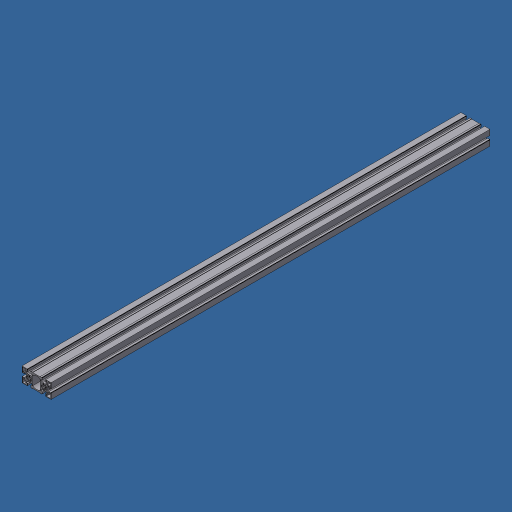
# Autodesk Inventor part: BAR, EXTRUDED ALUM, 45MMX90MM, BOSCH
Saved by Autodesk Inventor 2024.3 (Build 283343000, 343)
## iProperties
Manager: _
Category: _
Control State: 0
Master: False
Checked Out: False
Created: 2019-07-31
Checked By: 00
User Status: Work In Process
Material: Aluminum, 6061-T6
Description: BAR, EXTRUDED ALUM, 45MMX90MM, BOSCH
Document SubType Name: Modeling
Designer: -
Engr Approved By: R
Density: 2.71 g/cm^3
Mass: 5427.32 g
Surface Area: 13744.3 cm^2
Volume: 2002.7 cm^3
Mfg Approved By: -
Part Number: BAR, EXTRUDED ALUM, 45MMX90MM, BOSCH
Appearance: Aluminum (Flat)
Shininess: 64.0
Angle Display Precision: 2
Document Length Units: 11269
Document Angle Units: 11279
Document Time Units: 11290
Document Mass Units: 11283
Document Length Units Precision: 3
Document Angle Units Precision: 2
ILogicPurgeVersion: 2.2.20.20
Density: 0.0
Volumn: 0.0
Area: 0.0
PropertySet Name: Model Information
CN_MASS: 15.74
CN_SERVICEABLE: _
CL_runCount: 0
FIRST_DESCRIPTION: _
SECOND_DESCRIPTION: _
THIRD_DESCRIPTION: _
ModelCat: Uncategorized
Revision Number: A
Subject: _
Author: -
Keywords: -
Autodesk Inventor part; units mm, degrees
ref_plane "YZ Plane" through (0, 0, 0) normal (1, 0, 0) x (0, 1, 0)
ref_plane "XZ Plane" through (0, 0, 0) normal (0, 1, 0) x (-1, 0, 0)
ref_plane "XY Plane" through (0, 0, 0) normal (0, 0, 1) x (1, 0, 0)
sketch "Sketch1" plane through (0, 0, 0) normal (0, 0, 1) x (1, 0, 0)
  line L0 (0.8723, 4.7995) -> (0.562, 7.7834)
  line L1 (-0.9902, 4.2192) -> (-2.4189, 6.8572)
  line L2 (-2.4889, 2.9702) -> (-4.8184, 4.8607)
  line L3 (-3.3956, 1.2428) -> (-6.2711, 2.0979)
  line L4 (-3.5722, -0.7001) -> (-6.5561, -1.0105)
  line L5 (-2.9918, -2.5627) -> (-5.6298, -3.9913)
  line L6 (-1.7429, -4.0614) -> (-3.6333, -6.3908)
  line L7 (-0.0155, -4.9681) -> (-0.8706, -7.8436)
  line L8 (1.9274, -5.1447) -> (2.2378, -8.1286)
  line L9 (3.79, -4.5643) -> (5.2187, -7.2023)
  line L10 (5.2887, -3.3153) -> (7.6181, -5.2058)
  line L11 (6.1954, -1.5879) -> (9.0709, -2.443)
  line L12 (6.372, 0.355) -> (9.3559, 0.6654)
  line L13 (5.7916, 2.2176) -> (8.4296, 3.6462)
  line L14 (4.5427, 3.7163) -> (6.4331, 6.0457)
  line L15 (2.8152, 4.6229) -> (3.6704, 7.4985)
  arc A0 (-2.4889, 2.9702) -> (-3.3956, 1.2428) centre (1.3999, -0.1726) ccw
  arc A1 (-3.5722, -0.7001) -> (-2.9918, -2.5627) centre (1.3999, -0.1726) ccw
  arc A2 (-1.7429, -4.0614) -> (-0.0155, -4.9681) centre (1.3999, -0.1726) ccw
  arc A3 (1.9274, -5.1447) -> (3.79, -4.5643) centre (1.3999, -0.1726) ccw
  arc A4 (5.2887, -3.3153) -> (6.1954, -1.5879) centre (1.3999, -0.1726) ccw
  arc A5 (6.372, 0.355) -> (5.7916, 2.2176) centre (1.3999, -0.1726) ccw
  arc A6 (4.5427, 3.7163) -> (2.8152, 4.6229) centre (1.3999, -0.1726) ccw
  arc A7 (0.8723, 4.7995) -> (-0.9902, 4.2192) centre (1.3999, -0.1726) ccw
  arc A8 (8.4296, 3.6462) -> (6.4331, 6.0457) centre (1.3999, -0.1726) ccw
  arc A9 (9.0709, -2.443) -> (9.3559, 0.6654) centre (1.3999, -0.1726) ccw
  arc A10 (5.2187, -7.2023) -> (7.6181, -5.2058) centre (1.3999, -0.1726) ccw
  arc A11 (-0.8706, -7.8436) -> (2.2378, -8.1286) centre (1.3999, -0.1726) ccw
  arc A12 (-5.6298, -3.9913) -> (-3.6333, -6.3908) centre (1.3999, -0.1726) ccw
  arc A13 (-6.2711, 2.0979) -> (-6.5561, -1.0105) centre (1.3999, -0.1726) ccw
  arc A14 (3.6704, 7.4985) -> (0.562, 7.7834) centre (1.3999, -0.1726) ccw
  arc A15 (-2.4189, 6.8572) -> (-4.8184, 4.8607) centre (1.3999, -0.1726) ccw
  line L16 (-5.4014, 9.3274) -> (-1.7226, 9.3274)
  line L17 (4.5224, 9.3274) -> (8.0715, 9.3274)
  line L18 (8.2012, -9.6726) -> (4.5224, -9.6726)
  line L19 (-1.7226, -9.6726) -> (-5.2717, -9.6726)
  line L20 (-8.1001, -6.9739) -> (-8.1001, -3.2951)
  line L21 (-8.1001, 2.9499) -> (-8.1001, 6.499)
  arc A16 (-8.1001, 2.9499) -> (-8.1001, -3.2951) centre (1.3999, -0.1726) ccw
  arc A17 (4.5224, 9.3274) -> (-1.7226, 9.3274) centre (1.3999, -0.1726) ccw
  arc A18 (-1.7226, -9.6726) -> (4.5224, -9.6726) centre (1.3999, -0.1726) ccw
  line L22 (10.3005, 11.4268) -> (10.3005, 15.3274)
  line L23 (10.3005, 15.3274) -> (6.3999, 15.3274)
  line L24 (6.3999, 15.3274) -> (6.3999, 21.3274)
  line L25 (7.3999, 22.3274) -> (40.3999, 22.3274)
  line L26 (23.8999, 22.3274) -> (23.8999, 5.8274)
  line L27 (22.8999, 4.8274) -> (16.8999, 4.8274)
  line L28 (16.8999, 4.8274) -> (16.8999, 8.7281)
  line L29 (16.8999, 8.7281) -> (12.9992, 8.7281)
  line L30 (10.8999, 6.6287) -> (12.9992, 8.7281)
  line L31 (8.0715, 9.3274) -> (10.3005, 11.4268)
  line L32 (12.5715, 11.3425) -> (18.8822, 11.3425)
  line L33 (18.8822, 11.3425) -> (18.8822, 6.7953)
  line L34 (18.8822, 6.7953) -> (21.9064, 6.7953)
  line L35 (21.9064, 6.7953) -> (21.9064, 20.3274)
  line L36 (21.9064, 20.3274) -> (8.3743, 20.3274)
  line L37 (8.3743, 20.3274) -> (8.3743, 17.3032)
  line L38 (8.3743, 17.3032) -> (12.5715, 17.3032)
  line L39 (12.5715, 17.3032) -> (12.5715, 11.3425)
  line L40 (6.3999, 21.3274) -> (7.3999, 21.3274)
  line L41 (7.3999, 21.3274) -> (7.3999, 22.3274)
  line L42 (22.8999, 4.8274) -> (22.8999, 5.8274)
  line L43 (22.8999, 5.8274) -> (23.8999, 5.8274)
  line L44 (-10.1995, 8.7281) -> (-14.1001, 8.7281)
  line L45 (-14.1001, 8.7281) -> (-14.1001, 4.8274)
  line L46 (-14.1001, 4.8274) -> (-20.1001, 4.8274)
  line L47 (-21.1001, 5.8274) -> (-21.1001, 22.3274)
  line L48 (-21.1001, 22.3274) -> (-4.6001, 22.3274)
  line L49 (-3.6001, 21.3274) -> (-3.6001, 15.3274)
  line L50 (-3.6001, 15.3274) -> (-7.5008, 15.3274)
  line L51 (-7.5008, 15.3274) -> (-7.5008, 11.4268)
  line L52 (-5.4014, 9.3274) -> (-7.5008, 11.4268)
  line L53 (-8.1001, 6.499) -> (-10.1995, 8.7281)
  line L54 (-10.1152, 10.9991) -> (-10.1152, 17.3097)
  line L55 (-10.1152, 17.3097) -> (-5.568, 17.3097)
  line L56 (-5.568, 17.3097) -> (-5.568, 20.334)
  line L57 (-5.568, 20.334) -> (-19.1001, 20.334)
  line L58 (-19.1001, 20.334) -> (-19.1001, 6.8019)
  line L59 (-19.1001, 6.8019) -> (-16.0758, 6.8019)
  line L60 (-16.0758, 6.8019) -> (-16.0758, 10.9991)
  line L61 (-16.0758, 10.9991) -> (-10.1152, 10.9991)
  line L62 (-20.1001, 4.8274) -> (-20.1001, 5.8274)
  line L63 (-20.1001, 5.8274) -> (-21.1001, 5.8274)
  line L64 (-3.6001, 21.3274) -> (-4.6001, 21.3274)
  line L65 (-4.6001, 21.3274) -> (-4.6001, 22.3274)
  line L66 (-7.5008, -11.7719) -> (-7.5008, -15.6726)
  line L67 (-7.5008, -15.6726) -> (-3.6001, -15.6726)
  line L68 (-3.6001, -15.6726) -> (-3.6001, -21.6726)
  line L69 (-4.6001, -22.6726) -> (-21.1001, -22.6726)
  line L70 (-21.1001, -22.6726) -> (-21.1001, -6.1726)
  line L71 (-20.1001, -5.1726) -> (-14.1001, -5.1726)
  line L72 (-14.1001, -5.1726) -> (-14.1001, -9.0732)
  line L73 (-14.1001, -9.0732) -> (-10.1995, -9.0732)
  line L74 (-8.1001, -6.9739) -> (-10.1995, -9.0732)
  line L75 (-5.2717, -9.6726) -> (-7.5008, -11.7719)
  line L76 (-9.7717, -11.6876) -> (-16.0824, -11.6876)
  line L77 (-16.0824, -11.6876) -> (-16.0824, -7.1405)
  line L78 (-16.0824, -7.1405) -> (-19.1067, -7.1405)
  line L79 (-19.1067, -7.1405) -> (-19.1067, -20.6726)
  line L80 (-19.1067, -20.6726) -> (-5.5746, -20.6726)
  line L81 (-5.5746, -20.6726) -> (-5.5746, -17.6483)
  line L82 (-5.5746, -17.6483) -> (-9.7717, -17.6483)
  line L83 (-9.7717, -17.6483) -> (-9.7717, -11.6876)
  line L84 (-3.6001, -21.6726) -> (-4.6001, -21.6726)
  line L85 (-4.6001, -21.6726) -> (-4.6001, -22.6726)
  line L86 (-20.1001, -5.1726) -> (-20.1001, -6.1726)
  line L87 (-20.1001, -6.1726) -> (-21.1001, -6.1726)
  line L88 (12.9992, -9.0732) -> (16.8999, -9.0732)
  line L89 (16.8999, -9.0732) -> (16.8999, -5.1726)
  line L90 (16.8999, -5.1726) -> (22.8999, -5.1726)
  line L91 (23.8999, -6.1726) -> (23.8999, -22.6726)
  line L92 (40.3999, -22.6726) -> (7.3999, -22.6726)
  line L93 (6.3999, -21.6726) -> (6.3999, -15.6726)
  line L94 (6.3999, -15.6726) -> (10.3005, -15.6726)
  line L95 (10.3005, -15.6726) -> (10.3005, -11.7719)
  line L96 (8.2012, -9.6726) -> (10.3005, -11.7719)
  line L97 (10.8999, -6.8441) -> (12.9992, -9.0732)
  line L98 (12.9149, -11.3442) -> (12.9149, -17.6548)
  line L99 (12.9149, -17.6548) -> (8.3678, -17.6548)
  line L100 (8.3678, -17.6548) -> (8.3678, -20.6791)
  line L101 (8.3678, -20.6791) -> (21.8999, -20.6791)
  line L102 (21.8999, -20.6791) -> (21.8999, -7.147)
  line L103 (21.8999, -7.147) -> (18.8756, -7.147)
  line L104 (18.8756, -7.147) -> (18.8756, -11.3442)
  line L105 (18.8756, -11.3442) -> (12.9149, -11.3442)
  line L106 (22.8999, -5.1726) -> (22.8999, -6.1726)
  line L107 (22.8999, -6.1726) -> (23.8999, -6.1726)
  line L108 (6.3999, -21.6726) -> (7.3999, -21.6726)
  line L109 (7.3999, -21.6726) -> (7.3999, -22.6726)
  line L110 (46.9274, 4.7995) -> (47.2378, 7.7834)
  line L111 (48.79, 4.2192) -> (50.2187, 6.8572)
  line L112 (50.2887, 2.9702) -> (52.6181, 4.8607)
  line L113 (51.1954, 1.2428) -> (54.0709, 2.0979)
  line L114 (51.372, -0.7001) -> (54.3559, -1.0105)
  line L115 (50.7916, -2.5627) -> (53.4296, -3.9913)
  line L116 (49.5427, -4.0614) -> (51.4331, -6.3908)
  line L117 (47.8152, -4.9681) -> (48.6704, -7.8436)
  line L118 (45.8723, -5.1447) -> (45.562, -8.1286)
  line L119 (44.0098, -4.5643) -> (42.5811, -7.2023)
  line L120 (42.5111, -3.3153) -> (40.1816, -5.2058)
  line L121 (41.6044, -1.5879) -> (38.7289, -2.443)
  line L122 (41.4278, 0.355) -> (38.4439, 0.6654)
  line L123 (42.0082, 2.2176) -> (39.3702, 3.6462)
  line L124 (43.2571, 3.7163) -> (41.3667, 6.0457)
  line L125 (44.9845, 4.6229) -> (44.1294, 7.4985)
  arc A19 (51.1954, 1.2428) -> (50.2887, 2.9702) centre (46.3999, -0.1726) ccw
  arc A20 (50.7916, -2.5627) -> (51.372, -0.7001) centre (46.3999, -0.1726) ccw
  arc A21 (47.8152, -4.9681) -> (49.5427, -4.0614) centre (46.3999, -0.1726) ccw
  arc A22 (44.0098, -4.5643) -> (45.8723, -5.1447) centre (46.3999, -0.1726) ccw
  arc A23 (41.6044, -1.5879) -> (42.5111, -3.3153) centre (46.3999, -0.1726) ccw
  arc A24 (42.0082, 2.2176) -> (41.4278, 0.355) centre (46.3999, -0.1726) ccw
  arc A25 (44.9845, 4.6229) -> (43.2571, 3.7163) centre (46.3999, -0.1726) ccw
  arc A26 (48.79, 4.2192) -> (46.9274, 4.7995) centre (46.3999, -0.1726) ccw
  arc A27 (41.3667, 6.0457) -> (39.3702, 3.6462) centre (46.3999, -0.1726) ccw
  arc A28 (38.4439, 0.6654) -> (38.7289, -2.443) centre (46.3999, -0.1726) ccw
  arc A29 (40.1816, -5.2058) -> (42.5811, -7.2023) centre (46.3999, -0.1726) ccw
  arc A30 (45.562, -8.1286) -> (48.6704, -7.8436) centre (46.3999, -0.1726) ccw
  arc A31 (51.4331, -6.3908) -> (53.4296, -3.9913) centre (46.3999, -0.1726) ccw
  arc A32 (54.3559, -1.0105) -> (54.0709, 2.0979) centre (46.3999, -0.1726) ccw
  arc A33 (47.2378, 7.7834) -> (44.1294, 7.4985) centre (46.3999, -0.1726) ccw
  arc A34 (52.6181, 4.8607) -> (50.2187, 6.8572) centre (46.3999, -0.1726) ccw
  line L126 (53.2012, 9.3274) -> (49.5224, 9.3274)
  line L127 (49.5224, -9.6726) -> (53.0715, -9.6726)
  line L128 (55.8999, -6.9739) -> (55.8999, -3.2951)
  line L129 (55.8999, 2.9499) -> (55.8999, 6.499)
  arc A35 (55.8999, -3.2951) -> (55.8999, 2.9499) centre (46.3999, -0.1726) ccw
  arc A36 (49.5224, 9.3274) -> (43.2774, 9.3274) centre (46.3999, -0.1726) ccw
  arc A37 (43.2774, -9.6726) -> (49.5224, -9.6726) centre (46.3999, -0.1726) ccw
  line L130 (57.9992, 8.7281) -> (61.8999, 8.7281)
  line L131 (63.8756, 10.9991) -> (57.9149, 10.9991)
  line L132 (57.9149, 10.9991) -> (57.9149, 17.3097)
  line L133 (66.8999, 20.334) -> (66.8999, 6.8019)
  line L134 (68.8999, 5.8274) -> (68.8999, 22.3274)
  line L135 (61.8999, 8.7281) -> (61.8999, 4.8274)
  line L136 (61.8999, 4.8274) -> (67.8999, 4.8274)
  line L137 (63.8756, 6.8019) -> (63.8756, 10.9991)
  line L138 (66.8999, 6.8019) -> (63.8756, 6.8019)
  line L139 (67.8999, 5.8274) -> (68.8999, 5.8274)
  line L140 (67.8999, 4.8274) -> (67.8999, 5.8274)
  line L141 (53.3678, 20.334) -> (66.8999, 20.334)
  line L142 (68.8999, 22.3274) -> (52.3999, 22.3274)
  line L143 (51.3999, 15.3274) -> (55.3005, 15.3274)
  line L144 (51.3999, 21.3274) -> (51.3999, 15.3274)
  line L145 (51.3999, 21.3274) -> (52.3999, 21.3274)
  line L146 (53.3678, 17.3097) -> (53.3678, 20.334)
  line L147 (52.3999, 21.3274) -> (52.3999, 22.3274)
  line L148 (57.9149, 17.3097) -> (53.3678, 17.3097)
  line L149 (53.2012, 9.3274) -> (55.3005, 11.4268)
  line L150 (55.3005, 15.3274) -> (55.3005, 11.4268)
  line L151 (55.8999, 6.499) -> (57.9992, 8.7281)
  line L152 (55.3005, -11.7719) -> (55.3005, -15.6726)
  line L153 (57.5715, -17.6483) -> (57.5715, -11.6876)
  line L154 (57.5715, -11.6876) -> (63.8822, -11.6876)
  line L155 (66.9064, -20.6726) -> (53.3743, -20.6726)
  line L156 (52.3999, -22.6726) -> (68.8999, -22.6726)
  line L157 (55.3005, -15.6726) -> (51.3999, -15.6726)
  line L158 (51.3999, -15.6726) -> (51.3999, -21.6726)
  line L159 (53.3743, -17.6483) -> (57.5715, -17.6483)
  line L160 (53.3743, -20.6726) -> (53.3743, -17.6483)
  line L161 (52.3999, -21.6726) -> (52.3999, -22.6726)
  line L162 (51.3999, -21.6726) -> (52.3999, -21.6726)
  line L163 (66.9064, -7.1405) -> (66.9064, -20.6726)
  line L164 (68.8999, -22.6726) -> (68.8999, -6.1726)
  line L165 (61.8999, -5.1726) -> (61.8999, -9.0732)
  line L166 (67.8999, -5.1726) -> (61.8999, -5.1726)
  line L167 (67.8999, -5.1726) -> (67.8999, -6.1726)
  line L168 (63.8822, -7.1405) -> (66.9064, -7.1405)
  line L169 (67.8999, -6.1726) -> (68.8999, -6.1726)
  line L170 (63.8822, -11.6876) -> (63.8822, -7.1405)
  line L171 (55.8999, -6.9739) -> (57.9992, -9.0732)
  line L172 (61.8999, -9.0732) -> (57.9992, -9.0732)
  line L173 (53.0715, -9.6726) -> (55.3005, -11.7719)
  line L174 (37.4992, 11.4268) -> (37.4992, 15.3274)
  line L175 (37.4992, 15.3274) -> (41.3999, 15.3274)
  line L176 (41.3999, 15.3274) -> (41.3999, 21.3274)
  line L177 (39.7283, 9.3274) -> (37.4992, 11.4268)
  line L178 (41.3999, 21.3274) -> (40.3999, 21.3274)
  line L179 (40.3999, 21.3274) -> (40.3999, 22.3274)
  line L180 (41.3999, -15.6726) -> (37.4992, -15.6726)
  line L181 (41.3999, -21.6726) -> (41.3999, -15.6726)
  line L182 (41.3999, -21.6726) -> (40.3999, -21.6726)
  line L183 (40.3999, -21.6726) -> (40.3999, -22.6726)
  line L184 (39.5986, -9.6726) -> (37.4992, -11.7719)
  line L185 (37.4992, -15.6726) -> (37.4992, -11.7719)
  line L186 (43.2774, 9.3274) -> (39.7283, 9.3274)
  line L187 (39.5986, -9.6726) -> (43.2774, -9.6726)
  point P0 (12.5887, 13.4964)
  point P1 (-12.2691, 11.0163)
  point P2 (-9.7889, -13.8416)
  point P3 (15.0689, -11.3614)
  point P4 (60.0689, 11.0163)
  dimension "d4" = 360
  dimension "d7" = 5
  dimension "d8" = 8
  dimension "d13" = 10
  dimension "d14" = 10
  dimension "d16" = 10
  dimension "d22" = 5
  dimension "d24" = 22.5
  dimension "d27" = 6
  dimension "d28" = 1
  dimension "d29" = 1
  dimension "d34" = 360
  dimension "d36" = 45
  dimension "d37" = 45
  dimension "d38" = 10
  dimension "d39" = 10
  dimension "d42" = 45
  constraints: 376 end point, 76 point on circle, 57 parallel, 38 centre point, 20 perpendicular, 6 equal length, 4 coincident, 2 horizontal, 234 other
  measures "d7" radius of A6
  measures "d8" radius of A15
  measures "d13" radius of A16
  measures "d14" radius of A17
  measures "d16" radius of A18
  measures "d22" distance from line of A8.centre L24
  measures "d24" distance from line of L25 A8.centre
  measures "d27" distance between parallel lines of L17 L23
  measures "d28" distance of L24.end L40.end
  measures "d29" distance of L40.end L25.start
  measures "d36" distance between parallel lines of L69 L48
  measures "d37" distance between parallel lines of L91 L70
  measures "d38" distance between parallel lines of L93 L68
  measures "d39" distance between parallel lines of L71 L46
  measures "d42" angle of L74 L20
extrude "BOSCH, 45X90" add sketch "Sketch1" along normal blind 1360 contours L16 A17 L17 L31 L22 L23 L24 L40 L41 L25 L179 L178 L176 L175 L174 L177 L186 A36 L126 L149 L150 L143 L144 L145 L147 L142 L134 L139 L140 L136 L135 L130 L151 L129 A35 L128 L171 L172 L165 L166 L167 L169 L164 L156 L161 L162 L158 L157 L152 L173 L127 A37 L187 L184 L185 L180 L181 L182 L183 L92 L109 L108 L93 L94 L95 L96 L18 A18 L19 L75 L66 L67 L68 L84 L85 L69 L70 L87 L86 L71 L72 L73 L74 L20 A16 L21 L53 L44 L45 L46 L62 L63 L47 L48 L65 L64 L49 L50 L51 L52 | L39 L38 L37 L36 L35 L34 L33 L32 | L105 L104 L103 L102 L101 L100 L99 L98
sketch "Sketch2" plane through (0, 0, 1360) normal (0, 0, 1) x (1, 0, 0)
  line L0 (10.3005, 11.4268) -> (10.3005, 15.3274) projected
  line L1 (37.4992, -11.7719) -> (37.4992, -15.6726) projected
  line L2 (37.4992, 15.3274) -> (37.4992, 11.4268) projected
  line L3 (10.3005, -15.6726) -> (10.3005, -11.7719) projected
  line L4 (10.3005, 11.4268) -> (37.4992, -11.7719) construction
  line L5 (10.3005, -11.7719) -> (37.4992, 11.4268) construction
  line L6 (12.2563, 13.5543) -> (12.2563, -13.8995)
  line L7 (35.5434, 13.5543) -> (35.5434, -13.8995)
  arc A0 (12.2563, -13.8995) -> (35.5434, -13.8995) centre (23.8999, -0.1726) ccw
  arc A1 (35.5434, 13.5543) -> (12.2563, 13.5543) centre (23.8999, -0.1726) ccw
  line L8 (40.3999, -22.6726) -> (7.3999, -22.6726) projected
  line L9 (41.3999, -21.6726) -> (40.3999, -21.6726) projected
  line L10 (40.3999, 21.3274) -> (41.3999, 21.3274) projected
  line L11 (7.3999, 22.3274) -> (40.3999, 22.3274) projected
  line L12 (12.2563, 22.3274) -> (12.2563, 21.3274)
  line L13 (12.2563, 21.3274) -> (35.5434, 21.3274)
  line L14 (35.5434, 21.3274) -> (35.5434, 22.3274)
  line L15 (12.2563, -22.6726) -> (12.2563, -21.6726)
  line L16 (12.2563, -21.6726) -> (35.5434, -21.6726)
  line L17 (35.5434, -21.6726) -> (35.5434, -22.6726)
  dimension "d45" = 1.9558
  dimension "d46" = 1.9558
  dimension "d49" = 18
  dimension "d50" = 18
  constraints: 20 end point, 6 collinear, 4 parallel, 4 point on circle, 4 point on line, 3 perpendicular, 2 centre point, 1 midpoint
  measures "d45" distance between parallel lines of L2 L7
  measures "d46" distance between parallel lines of L0 L6
  measures "d49" radius of A0
  measures "d50" radius of A1
extrude "Extrusion2" cut sketch "Sketch2" against normal through all
sketch "Sketch7" plane through (-21.1001, -22.6726, 0) normal (0, -1, 0) x (1, 0, 0)
  line L0 (0, 0) -> (0, 1360) projected
  line L1 (16.5, 0) -> (16.5, 1360) projected
  line L2 (0, 680) -> (125.5103, 680)
  point P0 (22.5, 455)
  point P1 (22.5, 905)
  point P2 (67.5, 905)
  point P3 (67.5, 455)
  dimension "d110" = 450
  dimension "d111" = 225
  dimension "d112" = 22.5
  dimension "d113" = 45
  constraints: 2 end point, 2 horizontal alignment, 2 vertical alignment, 1 midpoint, 1 perpendicular
  measures "d110" distance of point (22.5, 455) point (22.5, 905)
  measures "d111" distance from line of point (22.5, 905) L2
  measures "d112" distance from line of point (22.5, 905) L0
  measures "d113" distance of point (67.5, 905) point (22.5, 905)
hole "Hole5" at (1.3999, -22.6726, 455) at (1.3999, -22.6726, 905) at (46.3999, -22.6726, 905) at (46.3999, -22.6726, 455) direction (0, 1, 0) diameter 9 end through all
equation "\"d14\" = d13"
equation "\"d16\" = d13"
equation "\"d22\" = d21"
equation "\"d27\" = d26"
equation "\"d29\" = d28"
equation "\"d50\" = d49"
equation "\"d111\" = 0.5 * d110"
equation "\"d10\" = d9"
equation "\"d11\" = d10"
equation "\"d21\" = 5"
equation "\"d26\" = 6"
equation "\"d9\" = 9.5"
